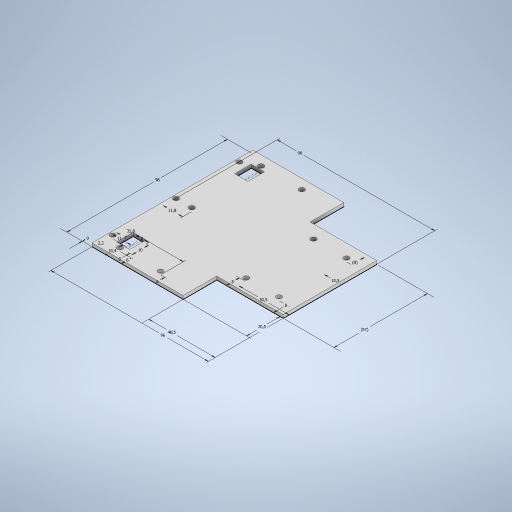
# Autodesk Inventor part: PodstawaPEM
Saved by Autodesk Inventor 2023 (Build 270158000, 158)
## iProperties
Created: 2023-01-05
Part Number: PodstawaPEM
Material: Ogólny
Document SubType Name: Modeling
Designer: mt150
Density: 1 g/cm^3
Appearance: Domyślna
Author: mt150
Autodesk Inventor part; units mm, degrees
ref_plane "YZ Plane" through (0, 0, 0) normal (1, 0, 0) x (0, 1, 0)
ref_plane "XZ Plane" through (0, 0, 0) normal (0, 1, 0) x (-1, 0, 0)
ref_plane "XY Plane" through (0, 0, 0) normal (0, 0, 1) x (1, 0, 0)
sketch "Szkic1" plane through (0, 0, 0) normal (0, 1, 0) x (-1, 0, 0)
  line L0 (40.5, 0) -> (96, 0)
  line L1 (96, 0) -> (96, -98)
  line L2 (96, -98) -> (40.5, -98)
  line L3 (0, -77.5) -> (0, -20.5)
  line L4 (40.5, 0) -> (40.5, -20.5)
  line L5 (40.5, -20.5) -> (0, -20.5)
  line L6 (40.5, -98) -> (40.5, -77.5)
  line L7 (40.5, -77.5) -> (0, -77.5)
  line L8 (0, -49) -> (96, -49) construction
  line L9 (10.5, -77.5) -> (10.5, -20.5) construction
  line L10 (30.5, -77.5) -> (30.5, -20.5) construction
  line L11 (93.8, 0) -> (93.8, -98) construction
  line L12 (96, -6) -> (40.5, -6) construction
  line L13 (96, -92) -> (40.5, -92) construction
  line L14 (84.2, 0) -> (84.2, -98) construction
  line L15 (85, 0) -> (85, -98) construction
  line L16 (89, -8) -> (81, -8)
  line L17 (81, -8) -> (81, -18)
  line L18 (81, -18) -> (89, -18)
  line L19 (89, -18) -> (89, -8)
  line L20 (89, -90) -> (81, -90)
  line L21 (81, -90) -> (81, -80)
  line L22 (81, -80) -> (89, -80)
  line L23 (89, -80) -> (89, -90)
  point P0 (0, 0)
  point P1 (30.5, -28.5)
  point P2 (30.5, -69.5)
  point P3 (10.5, -28.5)
  point P4 (10.5, -69.5)
  point P5 (93.8, -10.4)
  point P6 (93.8, -87.6)
  point P7 (93.8, -49)
  point P8 (60.2, -6)
  point P9 (60.2, -92)
  point P10 (84.2, -49)
  point P11 (85, -6)
  point P12 (85, -92)
  dimension "d0" = 98
  dimension "d2" = 20.5
  dimension "d3" = 40.5
  dimension "d12" = 96
  dimension "d42" = 57
  dimension "d71" = 10.4
  dimension "d72" = 6
  dimension "d73" = 2.2
  dimension "d81" = 35.8
  dimension "d89" = 30.5
  dimension "d90" = 8
  dimension "d91" = 8
  dimension "d92" = 8
  dimension "d93" = 11.8
  dimension "d94" = 11
  dimension "d95" = 10.5
  dimension "d96" = 6
  dimension "d97" = 0
  dimension "d98" = 96
  dimension "d106" = 8
  dimension "d107" = 10
  dimension "d108" = 7
  dimension "d109" = 8
  constraints: 48 end point, 18 point on line, 11 symmetric about line, 9 perpendicular, 5 parallel, 4 midpoint, 2 horizontal, 3 other
  measures "d0" distance of L0.end L1.end
  measures "d2" distance of L0.start L4.end
  measures "d3" distance of L3.end L4.end
  measures "d12" distance of L8.start L8.end
  measures "d42" distance of L3.start L3.end
  measures "d71" distance from line of L0 point (93.8, -10.4)
  measures "d72" distance from line of L0 point (60.2, -6)
  measures "d73" distance between parallel lines of L1 L11
  measures "d81" distance from line of L1 point (60.2, -6)
  measures "d89" distance between parallel lines of L3 L10
  measures "d90" distance from line of L5 point (10.5, -28.5)
  measures "d91" distance from line of L7 point (10.5, -69.5)
  measures "d92" distance from line of L5 point (30.5, -28.5)
  measures "d93" distance from line of L1 point (84.2, -49)
  measures "d94" distance between parallel lines of L1 L15
  measures "d95" distance between parallel lines of L3 L9
  measures "d96" distance from line of L0 point (85, -6)
  measures "d97" distance from line of point (0, 0) L0
  measures "d98" distance from line of point (0, 0) L1
  measures "d106" distance of L18.end L17.end
  measures "d107" distance of L17.end L16.end
  measures "d108" distance between parallel lines of L1 L19
  measures "d109" distance between parallel lines of L0 L16
extrude "Wyciągnięcie proste1" add sketch "Szkic1" along normal blind 2 contours L0 L1 L2 L6 L7 L3 L5 L4 | L19 L18 L17 L16 | L20 L21 L22 L23
hole "Hole4" at (-30.5, 0, -28.5) at (-30.5, 0, -69.5) at (-10.5, 0, -28.5) at (-10.5, 0, -69.5) direction (0, 1, 0) diameter 3.2 depth 10
hole "Otwór5" at (-93.8, 0, -10.4) at (-93.8, 0, -87.6) at (-93.8, 0, -49) direction (0, 1, 0) diameter 3.2 end through all clearance for "Śruba ze łbem stożkowym ISO 2009/7046" size "M3" standard "ISO"
hole "Hole6" at (-60.2, 0, -6) at (-60.2, 0, -92) direction (0, 1, 0) diameter 3.2 depth 30 clearance for "Countersunk Flat Head Screw ISO 2009/7046" size "M3" standard "ISO"
hole "Hole7" at (-84.2, 0, -49) direction (0, 1, 0) diameter 3.2 depth 30 clearance for "Slotted Cheese Head Screw ISO 1207" size "M3" standard "ISO"
hole "Hole8" at (-85, 0, -6) at (-85, 0, -92) direction (0, 1, 0) diameter 3.4 end through all clearance for "Countersunk Flat Head Screw ISO 2009/7046" size "M3" standard "ISO"
extrude "Extrusion2" cut sketch "Szkic1" along normal blind 10 contours L19 L18 L17 L16 | L20 L21 L22 L23
